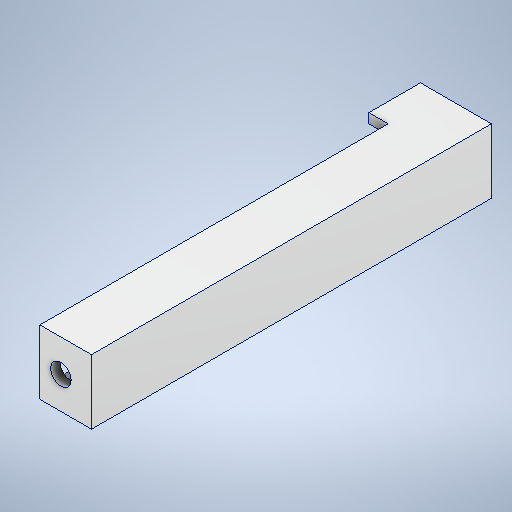
# Autodesk Inventor part: head_arm
Saved by Autodesk Inventor 2025 (Build 290162000, 162)
## iProperties
Created: 2024-04-25
Part Number: head_arm
Material: Hliník 6061
Document SubType Name: Modeling
Designer: rader
Density: 2.7 g/cm^3
Appearance: Hliník – plochý
Author: rader
Autodesk Inventor part; units mm, degrees
ref_plane "YZ Plane" through (0, 0, 0) normal (1, 0, 0) x (0, 1, 0)
ref_plane "XZ Plane" through (0, 0, 0) normal (0, 1, 0) x (-1, 0, 0)
ref_plane "XY Plane" through (0, 0, 0) normal (0, 0, 1) x (1, 0, 0)
sketch "Náčrt1" plane through (0, 0, 0) normal (0, 1, 0) x (-1, 0, 0)
  line L0 (0, -2) -> (0, 12) projected
  line L1 (-1.6, 0) -> (9.6, 0) projected
  line L2 (8, 10) -> (0, 10)
  line L3 (0, 10) -> (0, 0)
  line L4 (0, 0) -> (8, 0)
  line L5 (8, 0) -> (8, 10)
  line L6 (8, 8.5) -> (1.5, 8.5)
  line L7 (1.5, 8.5) -> (1.5, 1.5)
  line L8 (1.5, 1.5) -> (8, 1.5)
  line L9 (8, 1.5) -> (8, 8.5)
  point P0 (0, 0)
  point P1 (0, 10)
  dimension "d0" = 8
  dimension "d1" = 10
  dimension "d2" = 6.5
  dimension "d3" = 7
  dimension "d4" = 1.5
  constraints: 16 end point, 4 parallel, 2 collinear, 2 horizontal, 2 perpendicular, 1 point on line
  measures "d0" distance of L4.end L3.end
  measures "d1" distance of L3.end L2.end
  measures "d2" distance of L8.end L7.end
  measures "d3" distance of L7.end L6.end
  measures "d4" distance between parallel lines of L4 L8
extrude "Vysunutí1" add sketch "Náčrt1" along normal mid plane 59 contours L0 L2 L5 L6 L7 L8 L1
sketch "Náčrt2" plane through (0, -29.5, 0) normal (0, -1, 0) x (1, 0, 0)
  line L0 (-8, 8.5) -> (-1.5, 8.5) projected
  line L1 (-1.5, 8.5) -> (-1.5, 1.5) projected
  line L2 (-1.5, 1.5) -> (-8, 1.5) projected
  line L3 (-8, 1.5) -> (-8, 0) projected
  line L4 (-8, 0) -> (0, 0) projected
  line L5 (0, 0) -> (0, 10) projected
  line L6 (0, 10) -> (-8, 10) projected
  line L7 (-8, 10) -> (-8, 8.5) projected
  line L8 (-8, 10) -> (0, 10)
  line L9 (0, 10) -> (0, 0)
  line L10 (0, 0) -> (-8, 0)
  line L11 (-8, 0) -> (-8, 10)
  constraints: 8 end point, 2 parallel, 1 horizontal, 1 perpendicular
extrude "Vysunutí2" add sketch "Náčrt2" along normal blind 1.5
sketch "Náčrt3" plane through (0, -29.5, 0) normal (0, 1, 0) x (1, 0, 0)
  line L0 (-8, -8.5) -> (-1.5, -8.5) projected
  line L1 (-1.5, -8.5) -> (-1.5, -1.5) projected
  line L2 (-1.5, -1.5) -> (-8, -1.5) projected
  line L3 (-8, -8.5) -> (-8, -1.5) projected
  point P0 (0, 0)
  point P1 (-4.75, -5)
  dimension "d9" = 3.25
  dimension "d10" = 3.5
  measures "d9" distance from line of L3 point (-4.75, -5)
  measures "d10" distance from line of L0 point (-4.75, -5)
hole "Díra1" at (-4.75, -29.5, 5) direction (0, -1, 0) diameter 3.2 end through all
sketch "Náčrt5" plane through (0, 29.5, 0) normal (0, 1, 0) x (1, 0, 0)
  line L0 (0, -10) -> (-8, -10) projected
  line L1 (0, 0) -> (-8, 0)
  line L2 (-8, 0) -> (-8, -10)
  line L3 (-8, -10) -> (0, -10)
  line L4 (0, -10) -> (0, 0)
  constraints: 8 end point, 2 parallel, 1 horizontal, 1 perpendicular
extrude "Vysunutí3" add sketch "Náčrt5" along normal blind 1.5
sketch "Náčrt6" plane through (-8, -31, 0) normal (-1, 0, 0) x (0, 0, 1)
  line L0 (0, 0) -> (0, 62) projected
  line L1 (0, 62) -> (0, 54)
  line L2 (0, 54) -> (1.5, 54)
  line L3 (1.5, 1.5) -> (1.5, 60.5) projected
  line L4 (1.5, 60.5) -> (1.5, 54)
  line L5 (0, 0) -> (0, 62) projected
  line L6 (10, 0) -> (0, 0) projected
  line L7 (10, 0) -> (10, 62) projected
  line L8 (0, 62) -> (10, 62) projected
  line L9 (1.5, 60.5) -> (8.5, 60.5) projected
  line L10 (8.5, 1.5) -> (8.5, 60.5) projected
  line L11 (8.5, 1.5) -> (1.5, 1.5) projected
  line L12 (1.5, 1.5) -> (1.5, 60.5) projected
  line L13 (1.5, 60.5) -> (8.5, 60.5)
  line L14 (8.5, 60.5) -> (8.5, 54)
  line L15 (8.5, 60.5) -> (8.5, 1.5) projected
  line L16 (10, 54) -> (8.5, 54)
  line L17 (10, 54) -> (10, 62)
  line L18 (0, 62) -> (10, 62)
  point P0 (0, 31)
  dimension "d31" = 8
  dimension "d32" = 8
  constraints: 16 end point, 4 point on line, 3 collinear, 3 perpendicular
  measures "d31" distance of L0.end L1.end
  measures "d32" distance between parallel lines of L8 L16
extrude "Vysunutí4" add sketch "Náčrt6" along normal blind 3 contours L0 L8 L7 L16 L10 L9 L3 L2
sketch "Náčrt7" plane through (0, 31, 0) normal (0, 1, 0) x (1, 0, 0)
  line L0 (0, -10) -> (-11, -10) projected
  line L1 (0, -10) -> (0, 0) projected
  line L2 (0, 0) -> (-11, 0) projected
  line L3 (-11, -10) -> (-11, 0) projected
  point P0 (-2.5, -5)
  dimension "d35" = 2.5
  dimension "d37" = 5
  measures "d35" distance from line of L1 point (-2.5, -5)
  measures "d37" distance from line of L0 point (-2.5, -5)
hole "Díra3" at (-2.5, 31, 5) direction (0, -1, 0) diameter 1.5 depth 1.5
sketch "Náčrt8" plane through (0, 31, 0) normal (0, 1, 0) x (1, 0, 0)
  circle A0 centre (-2.5, -5) radius 0.75 projected
  line L0 (0, -10) -> (-11, -10) projected
  line L1 (0, -10) -> (0, 0) projected
  line L2 (0, 0) -> (-11, 0) projected
  line L3 (-11, -10) -> (-11, 0) projected
  point P0 (-8, -5)
  dimension "d45" = 3
  dimension "d46" = 5
  measures "d45" distance from line of L3 point (-8, -5)
  measures "d46" distance from line of L0 point (-8, -5)
hole "Díra4" at (-8, 31, 5) direction (0, -1, 0) diameter 3 depth 1.5
